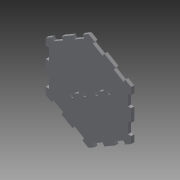
# Autodesk Inventor part: base
Saved by Autodesk Inventor 2015 (Build 190159000, 159)
## iProperties
Created: 2017-11-28
Part Number: base
Material: Generic
Document SubType Name: Modeling
Designer: Max
Density: 1 g/cm^3
Appearance: Default
Author: Max
Autodesk Inventor part; units mm, degrees
ref_plane "YZ Plane" through (0, 0, 0) normal (1, 0, 0) x (0, 1, 0)
ref_plane "XZ Plane" through (0, 0, 0) normal (0, 1, 0) x (-1, 0, 0)
ref_plane "XY Plane" through (0, 0, 0) normal (0, 0, 1) x (1, 0, 0)
sketch "Sketch1" plane through (0, 0, 0) normal (0, 1, 0) x (-1, 0, 0)
  line L0 (75.0098, 31.2127) -> (69.5098, 31.2127)
  line L1 (75.0098, 31.2127) -> (80.5098, 31.2127) construction
  line L2 (69.5098, 31.2127) -> (69.5098, 11.2127)
  line L3 (69.5098, 11.2127) -> (75.0098, 11.2127)
  line L4 (75.0098, -11.213) -> (69.5098, -11.213)
  line L5 (69.5098, -11.213) -> (69.5098, -31.213)
  line L6 (69.5098, -31.213) -> (75.0098, -31.213)
  line L7 (75.0098, -31.213) -> (75.0098, -43.3013)
  line L8 (75.0098, 43.3013) -> (75.0098, 31.2127)
  line L9 (75.0098, 11.2127) -> (75.0098, -11.213)
  line L10 (64.5408, -49.3456) -> (61.7908, -44.5824)
  line L11 (64.5408, -49.3456) -> (67.2908, -54.1087) construction
  line L12 (61.7908, -44.5824) -> (44.4702, -54.5824)
  line L13 (44.4702, -54.5824) -> (47.2202, -59.3456)
  line L14 (27.799, -70.5584) -> (25.049, -65.7953)
  line L15 (25.049, -65.7953) -> (7.7285, -75.7953)
  line L16 (7.7285, -75.7953) -> (10.4785, -80.5584)
  line L17 (10.4785, -80.5584) -> (0.0098, -86.6025)
  line L18 (75.0098, -43.3013) -> (64.5408, -49.3456)
  line L19 (47.2202, -59.3456) -> (27.799, -70.5584)
  line L20 (-10.4592, -80.5582) -> (-7.7092, -75.7951)
  line L21 (-10.4592, -80.5582) -> (-13.2092, -85.3214) construction
  line L22 (-7.7092, -75.7951) -> (-25.0298, -65.7951)
  line L23 (-25.0298, -65.7951) -> (-27.7798, -70.5582)
  line L24 (-47.201, -59.3454) -> (-44.451, -54.5823)
  line L25 (-44.451, -54.5823) -> (-61.7715, -44.5823)
  line L26 (-61.7715, -44.5823) -> (-64.5215, -49.3454)
  line L27 (-64.5215, -49.3454) -> (-74.9902, -43.3013)
  line L28 (0.0098, -86.6025) -> (-10.4592, -80.5582)
  line L29 (-27.7798, -70.5582) -> (-47.201, -59.3454)
  line L30 (-74.9902, -31.2127) -> (-69.4902, -31.2127)
  line L31 (-74.9902, -31.2127) -> (-80.4902, -31.2127) construction
  line L32 (-69.4902, -31.2127) -> (-69.4902, -11.2127)
  line L33 (-69.4902, -11.2127) -> (-74.9902, -11.2127)
  line L34 (-74.9902, 11.213) -> (-69.4902, 11.213)
  line L35 (-69.4902, 11.213) -> (-69.4902, 31.213)
  line L36 (-69.4902, 31.213) -> (-74.9902, 31.213)
  line L37 (-74.9902, 31.213) -> (-74.9902, 43.3013)
  line L38 (-74.9902, -43.3013) -> (-74.9902, -31.2127)
  line L39 (-74.9902, -11.2127) -> (-74.9902, 11.213)
  line L40 (-64.5212, 49.3456) -> (-61.7712, 44.5824)
  line L41 (-64.5212, 49.3456) -> (-67.2712, 54.1087) construction
  line L42 (-61.7712, 44.5824) -> (-44.4507, 54.5824)
  line L43 (-44.4507, 54.5824) -> (-47.2007, 59.3456)
  line L44 (-27.7795, 70.5584) -> (-25.0295, 65.7953)
  line L45 (-25.0295, 65.7953) -> (-7.709, 75.7953)
  line L46 (-7.709, 75.7953) -> (-10.459, 80.5584)
  line L47 (-10.459, 80.5584) -> (0.0098, 86.6025)
  line L48 (-74.9902, 43.3013) -> (-64.5212, 49.3456)
  line L49 (-47.2007, 59.3456) -> (-27.7795, 70.5584)
  line L50 (10.4788, 80.5582) -> (7.7288, 75.7951)
  line L51 (10.4788, 80.5582) -> (13.2288, 85.3214) construction
  line L52 (7.7288, 75.7951) -> (25.0493, 65.7951)
  line L53 (25.0493, 65.7951) -> (27.7993, 70.5582)
  line L54 (47.2205, 59.3454) -> (44.4705, 54.5823)
  line L55 (44.4705, 54.5823) -> (61.791, 44.5823)
  line L56 (61.791, 44.5823) -> (64.541, 49.3454)
  line L57 (64.541, 49.3454) -> (75.0098, 43.3013)
  line L58 (0.0098, 86.6025) -> (10.4788, 80.5582)
  line L59 (27.7993, 70.5582) -> (47.2205, 59.3454)
  line L60 (64.541, 49.3454) -> (75.0098, 43.3013)
  line L61 (0.0098, 86.6025) -> (10.4788, 80.5582)
  line L62 (27.7993, 70.5582) -> (47.2205, 59.3454)
  line L63 (-10.459, 80.5584) -> (0.0098, 86.6025)
  line L64 (-74.9902, 43.3013) -> (-64.5212, 49.3456)
  line L65 (-47.2007, 59.3456) -> (-27.7795, 70.5584)
  line L66 (-74.9902, 31.213) -> (-74.9902, 43.3013)
  line L67 (-74.9902, -43.3013) -> (-74.9902, -31.2127)
  line L68 (-74.9902, -11.2127) -> (-74.9902, 11.213)
  line L69 (-64.5215, -49.3454) -> (-74.9902, -43.3013)
  line L70 (0.0098, -86.6025) -> (-10.4592, -80.5582)
  line L71 (-27.7798, -70.5582) -> (-47.201, -59.3454)
  line L72 (10.4785, -80.5584) -> (0.0098, -86.6025)
  line L73 (75.0098, -43.3013) -> (64.5408, -49.3456)
  line L74 (47.2202, -59.3456) -> (27.799, -70.5584)
  point P0 (0.0098, 0)
  point P1 (0.0098, 0)
  point P2 (0.0098, 0)
  point P3 (0.0098, 0)
  point P4 (0.0098, 0)
  point P5 (0.0098, 0)
  dimension "d6" = 86.6025
  dimension "d7" = 5.5
  dimension "d8" = 180
  dimension "d9" = 20
  dimension "d10" = 20
  dimension "d13" = 360
  constraints: 150 end point, 11 perpendicular, 2 coincident, 2 horizontal, 1 collinear, 137 other
  measures "d6" distance of L8.start L7.end
  measures "d7" distance of L0.start L0.end
  measures "d8" angle of L0 L1
  measures "d9" distance of L0.end L2.end
  measures "d10" distance of L4.end L5.end
extrude "Extrusion1" add sketch "Sketch1" along normal blind 5.5
sketch "Sketch2" plane through (0, 0, 0) normal (0, -1, 0) x (1, 0, 0)
  line L0 (-17.3205, -10) -> (-25.9808, -15)
  line L1 (-25.9808, -15) -> (-24.9808, -16.7321)
  line L2 (-24.9808, -16.7321) -> (-16.3205, -11.7321)
  line L3 (-16.3205, -11.7321) -> (-17.3205, -10)
  line L4 (17.3205, 10) -> (25.9808, 15)
  line L5 (25.9808, 15) -> (26.9808, 13.2679)
  line L6 (26.9808, 13.2679) -> (18.3205, 8.2679)
  line L7 (18.3205, 8.2679) -> (17.3205, 10)
  point P0 (0, 0)
  dimension "d17" = 10
  dimension "d18" = 2
  dimension "d19" = 10
  dimension "d22" = 20
  dimension "d23" = 20
  constraints: 16 end point, 4 parallel, 2 perpendicular
  measures "d17" distance of L2.end L1.end
  measures "d18" distance of L1.end L0.end
  measures "d19" distance of L5.end L6.end
  measures "d22" distance from line of L7 point (0, 0)
  measures "d23" distance from line of point (0, 0) L3
extrude "Extrusion2" cut sketch "Sketch2" against normal blind 10
sketch "Sketch4" plane through (0, 0, 0) normal (0, -1, 0) x (1, 0, 0)
  line L0 (13.9904, 5.7679) -> (9.6603, 3.2679)
  line L1 (9.6603, 3.2679) -> (12.4103, -1.4952)
  line L2 (12.4103, -1.4952) -> (16.7404, 1.0048)
  line L3 (16.7404, 1.0048) -> (13.9904, 5.7679)
  line L4 (31.3109, 15.7679) -> (35.641, 18.2679)
  line L5 (35.641, 18.2679) -> (38.391, 13.5048)
  line L6 (38.391, 13.5048) -> (34.0609, 11.0048)
  line L7 (34.0609, 11.0048) -> (31.3109, 15.7679)
  line L8 (-11.9904, -9.2321) -> (-7.6603, -6.7321)
  line L9 (-7.6603, -6.7321) -> (-4.9103, -11.4952)
  line L10 (-4.9103, -11.4952) -> (-9.2404, -13.9952)
  line L11 (-9.2404, -13.9952) -> (-11.9904, -9.2321)
  line L12 (-29.3109, -19.2321) -> (-33.641, -21.7321)
  line L13 (-33.641, -21.7321) -> (-30.891, -26.4952)
  line L14 (-30.891, -26.4952) -> (-26.5609, -23.9952)
  line L15 (-26.5609, -23.9952) -> (-29.3109, -19.2321)
  point P0 (0, 0)
  dimension "d24" = 5
  dimension "d25" = 5.5
  dimension "d26" = 5
  dimension "d27" = 5.5
  constraints: 32 end point, 4 parallel, 2 perpendicular, 2 point on line
  measures "d24" distance of L2.end L1.end
  measures "d25" distance of L1.end L0.end
  measures "d26" distance of L5.end L6.end
  measures "d27" distance of L4.end L5.end
extrude "Extrusion3" cut sketch "Sketch4" against normal blind 10
body "Solid1"
